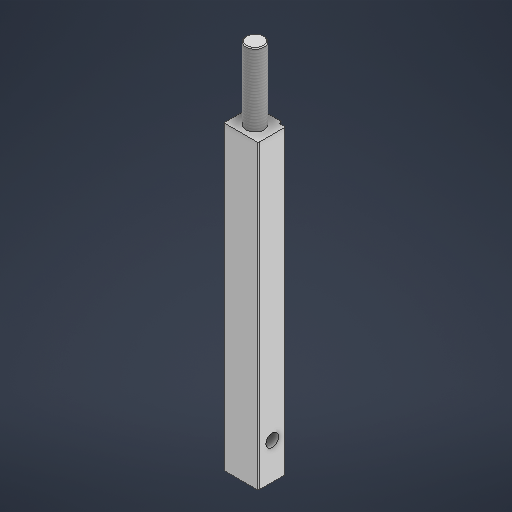
# Autodesk Inventor part: oszlop
Saved by Autodesk Inventor 2026.1 (Build 301233000, 233)
## iProperties
Created: 2025-09-15
Part Number: oszlop
Material: Generic
Document SubType Name: Modeling
Designer: student
Density: 1 g/cm^3
Appearance: Default
Author: student
Autodesk Inventor part; units mm, degrees
ref_plane "YZ Plane" through (0, 0, 0) normal (1, 0, 0) x (0, 1, 0)
ref_plane "XZ Plane" through (0, 0, 0) normal (0, 1, 0) x (-1, 0, 0)
ref_plane "XY Plane" through (0, 0, 0) normal (0, 0, 1) x (1, 0, 0)
sketch "Sketch1" plane through (0, 0, 0) normal (0, 1, 0) x (-1, 0, 0)
  line L0 (-9.5, 8.25) -> (9.5, 8.25)
  line L1 (9.5, 8.25) -> (9.5, -8.25)
  line L2 (9.5, -8.25) -> (-9.5, -8.25)
  line L3 (-9.5, -8.25) -> (-9.5, 8.25)
  line L4 (-9.5, 8.25) -> (9.5, -8.25) construction
  line L5 (9.5, 8.25) -> (-9.5, -8.25) construction
  line L6 (-6, 6.75) -> (6, 6.75)
  line L7 (6, 6.75) -> (6, -6.75)
  line L8 (6, -6.75) -> (-6, -6.75)
  line L9 (-6, -6.75) -> (-6, 6.75)
  line L10 (-6, 6.75) -> (6, -6.75) construction
  line L11 (6, 6.75) -> (-6, -6.75) construction
  line L12 (6, -6.75) -> (9.5, -6.75)
  line L13 (-6, -6.75) -> (-9.7082, -6.75)
  line L14 (6, -6.75) -> (6, -8.25)
  line L15 (-6, -6.75) -> (-6, -8.25)
  point P0 (0, 0)
  point P1 (-9.5, -6.75)
  dimension "d0" = 19
  dimension "d1" = 16.5
  dimension "d2" = 12
  dimension "d3" = 1.5
  constraints: 32 end point, 5 perpendicular, 4 midpoint, 4 parallel, 4 point on line, 2 horizontal
  measures "d0" distance of L1.end L2.end
  measures "d1" distance of L0.end L1.end
  measures "d2" distance of L7.end L8.end
  measures "d3" distance between parallel lines of L2 L8
extrude "Extrusion1" add sketch "Sketch1" along normal blind 166 contours L0 L1 L12 L7 L6 L9 L13 L3 | L9 L6 L7 L8 | L8 L14 L2 L15
sketch "Sketch2" plane through (0, 166, 0) normal (0, 1, 0) x (1, 0, 0)
  line L0 (-9.5, -8.25) -> (9.5, -8.25) projected
  line L1 (9.5, -8.25) -> (0, -8.25)
  line L2 (0, -8.25) -> (0, -0.5)
  line L3 (0, -0.5) -> (9.5, -0.5)
  line L4 (9.5, -0.5) -> (9.5, -8.25)
  circle A0 centre (0, -0.5) radius 5
  point P0 (0, 0)
  dimension "d6" = 7.75
  dimension "d7" = 10
  constraints: 8 end point, 2 parallel, 1 centre point, 1 coincident, 1 horizontal, 1 perpendicular
  measures "d6" distance of L1.end L2.end
  measures "d7" diameter of A0
extrude "Extrusion2" add sketch "Sketch2" along normal blind 40 contours A0 L3 L2 | L2 L3 A0
thread "Thread1" size "M10x1.5" class "6g" standard "ANSI Metric M Profile" length 40
chamfer "Chamfer1" distance 0.5 angle 45 1 edges at (-5, 206, 0.5)
fillet "Fillet1" radius 0.5 8 edges at (9.5, 83, -6.75) (6, 83, -8.25) (9.5, 83, 8.25) (-9.5, 83, 8.25) (-9.5, 83, -6.75) (-6, 83, -6.75) (-6, 83, -8.25) (6, 83, -6.75)
sketch "Sketch3" plane through (-9.5, 0, -6.25) normal (-1, 0, 0) x (0, 0, 1)
  line L0 (14.5, 0) -> (14.5, 166) projected
  line L1 (14.5, 0) -> (6.75, 0)
  line L2 (6.75, 0) -> (6.75, 206.1896)
  line L3 (6.75, 206.1896) -> (14.5, 206.1896)
  line L4 (14.5, 206.1896) -> (14.5, 0)
  line L5 (6.75, 0) -> (6.75, 20)
  circle A0 centre (6.75, 20) radius 3.5
  point P0 (6.25, 0)
  dimension "d16" = 20
  dimension "d17" = 7
  constraints: 10 end point, 2 parallel, 1 centre point, 1 coincident, 1 horizontal, 1 perpendicular, 1 point on line
  measures "d16" distance of L1.end L5.end
  measures "d17" diameter of A0
extrude "Extrusion3" cut sketch "Sketch3" against normal through all contours A0 L2 | L2 A0
body "Solid1"
